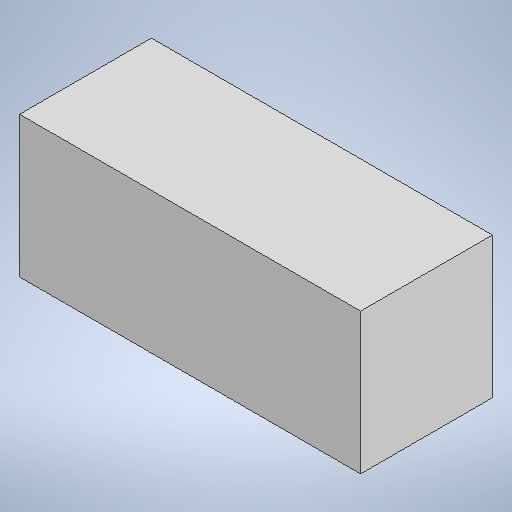
# Autodesk Inventor part: lily+gps
Saved by Autodesk Inventor 2025.3 (Build 293356000, 356)
## iProperties
Created: 2025-06-08
Part Number: lily+gps
Material: Generic
Document SubType Name: Modeling
Designer: Repete
Density: 1 g/cm^3
Appearance: Default
Author: Repete
Autodesk Inventor part; units mm, degrees
ref_plane "YZ Plane" through (0, 0, 0) normal (1, 0, 0) x (0, 1, 0)
ref_plane "XZ Plane" through (0, 0, 0) normal (0, 1, 0) x (-1, 0, 0)
ref_plane "XY Plane" through (0, 0, 0) normal (0, 0, 1) x (1, 0, 0)
sketch "Sketch1" plane through (0, 0, 0) normal (0, 1, 0) x (-1, 0, 0)
  line L0 (29.2308, 13.1026) -> (-45.7692, 13.1026)
  line L1 (-45.7692, 13.1026) -> (-45.7692, -17.8974)
  line L2 (-45.7692, -17.8974) -> (29.2308, -17.8974)
  line L3 (29.2308, -17.8974) -> (29.2308, 13.1026)
  point P0 (0, 0)
  dimension "d0" = 31
  dimension "d1" = 75
  constraints: 8 end point, 2 parallel, 1 horizontal, 1 perpendicular
  measures "d0" distance of L2.end L0.start
  measures "d1" distance of L1.end L2.end
extrude "Extrusion1" add sketch "Sketch1" along normal blind 29
body "Solid1"
